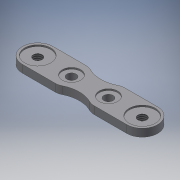
# Autodesk Inventor part: Tarot-mr4008-blade-adapter
Saved by Autodesk Inventor 2019.4 (Build 234330000, 330)
## iProperties
Created: 2019-06-24
Part Number: Tarot-mr4008-blade-adapter
Material: Generic
Document SubType Name: Modeling
Designer: cdi
Density: 1 g/cm^3
Appearance: Default
Author: cdi
Autodesk Inventor part; units mm, degrees
ref_plane "YZ Plane" through (0, 0, 0) normal (1, 0, 0) x (0, 1, 0)
ref_plane "XZ Plane" through (0, 0, 0) normal (0, 1, 0) x (-1, 0, 0)
ref_plane "XY Plane" through (0, 0, 0) normal (0, 0, 1) x (1, 0, 0)
sketch "Sketch1" plane through (0, 0, 0) normal (0, 1, 0) x (-1, 0, 0)
  line L0 (17, 5) -> (-17, 5)
  line L1 (-17, 5) -> (-17, -5)
  line L2 (-17, -5) -> (17, -5)
  line L3 (17, -5) -> (17, 5)
  line L4 (17, 5) -> (-17, -5) construction
  line L5 (-17, 5) -> (17, -5) construction
  point P0 (0, 0)
  dimension "d0" = 34
  dimension "d1" = 10
  constraints: 12 end point, 2 midpoint, 2 parallel, 1 horizontal, 1 perpendicular
  measures "d0" distance of L2.end L1.end
  measures "d1" distance of L0.end L1.end
extrude "Extrusion1" add sketch "Sketch1" along normal blind 2.5
sketch "Sketch2" plane through (0, 2.5, 0) normal (0, 1, 0) x (1, 0, 0)
  line L0 (-17, 5) -> (-17, -5) projected
  circle A0 centre (-17, 0) radius 5
  line L1 (17, -5) -> (17, 5) projected
  circle A1 centre (17, 0) radius 5
  point P0 (0, 0)
  constraints: 2 midpoint, 2 vertical alignment, 4 other
extrude "Extrusion2" add sketch "Sketch2" against normal blind 2.5
sketch "Sketch3" plane through (0, 2.5, 0) normal (0, 1, 0) x (1, 0, 0)
  arc A0 (-17, 5) -> (-17, -5) centre (-17, 0) ccw projected
  circle A1 centre (-17, 0) radius 1.5
  arc A2 (17, -5) -> (17, 5) centre (17, 0) ccw projected
  circle A3 centre (17, 0) radius 1.5
  point P0 (0, 0)
  dimension "d6" = 3
  dimension "d7" = 3
  constraints: 2 centre point, 2 coincident
  measures "d6" diameter of A1
  measures "d7" diameter of A3
hole "Hole1" at (-17, 2.5, 0) at (17, 2.5, 0) direction (0, -1, 0) diameter 2.85 end through all thread size "M3.5x0.6" class "6H" standard "ISO Metric profile"
sketch "Sketch4" plane through (0, 2.5, 0) normal (0, 1, 0) x (1, 0, 0)
  circle A0 centre (-17, 0) radius 4.25
  arc A1 (-17, 5) -> (-17, -5) centre (-17, 0) ccw projected
  arc A2 (17, -5) -> (17, 5) centre (17, 0) ccw projected
  circle A3 centre (17, 0) radius 4.25
  point P0 (0, 0)
  dimension "d15" = 8.5
  dimension "d16" = 8.5
  constraints: 2 centre point, 1 coincident, 1 concentric
  measures "d15" diameter of A0
  measures "d16" diameter of A3
extrude "Extrusion3" cut sketch "Sketch4" against normal blind 0.5
sketch "Sketch5" plane through (0, 2.5, 0) normal (0, 1, 0) x (1, 0, 0)
  circle A0 centre (0, 5) radius 1.5
  circle A1 centre (0, -5) radius 1.5
  circle A2 centre (0, 13.5) radius 10
  point P0 (0, 0)
  dimension "d19" = 3
  dimension "d20" = 5
  dimension "d21" = 3
  dimension "d22" = 5
  dimension "d23" = 20
  constraints: 3 centre point, 1 tangent
  measures "d19" diameter of A0
  measures "d20" distance of point (0, 0) A0.centre
  measures "d21" diameter of A1
  measures "d22" distance of point (0, 0) A1.centre
  measures "d23" diameter of A2
extrude "Extrusion4" cut sketch "Sketch5" against normal through all contours A0 | A2
mirror "Mirror1" about plane through (0, 0, 0) normal (0, 0, 1) of "Extrusion4"
sketch "Sketch6" plane through (0, 2.5, 0) normal (0, 1, 0) x (1, 0, 0)
  circle A0 centre (6, 0) radius 3
  point P0 (0, 0)
  dimension "d26" = 6
  dimension "d27" = 6
  constraints: 1 centre point
  measures "d26" diameter of A0
  measures "d27" distance of point (0, 0) A0.centre
extrude "Extrusion5" cut sketch "Sketch6" against normal blind 0.5
sketch "Sketch7" plane through (6, 2, 0) normal (0, 1, 0) x (1, 0, 0)
  circle A0 centre (0, 0) radius 3 projected
  circle A1 centre (0, 0) radius 1.5
  point P0 (-6, 0)
  dimension "d30" = 3
  constraints: 1 centre point, 1 coincident
  measures "d30" diameter of A1
extrude "Extrusion6" cut sketch "Sketch7" against normal through all contours A1
mirror "Mirror2" about plane through (0, 0, 0) normal (1, 0, 0) of "Extrusion5", "Extrusion6"
fillet "Fillet1" radius 4 4 edges at (5.2678, 1.25, 5) (-5.2678, 1.25, 5) (5.2678, 1.25, -5) (-5.2678, 1.25, -5)
body "Solid1"
